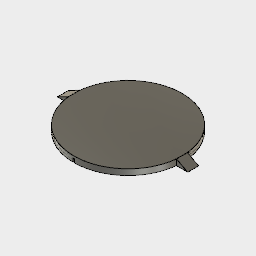
Sand Hopper Lid v1 (Autodesk Fusion 360 design; units mm, degrees)
Autodesk Fusion 360 part; units mm, degrees
sketch "Sketch1" plane through (0, 0, 0) normal (0, 0, 1) x (1, 0, 0)
  circle A0 centre (0, 0) radius 72.5
  dimension "d1" = 145
  constraint coincident A0.centre origin
  measures "d1" diameter of A0
extrude "Extrude1" add sketch "Sketch1" along normal blind 2
sketch "Sketch2" plane through (0, 0, 2) normal (0, 0, 1) x (-1, 0, 0)
  circle A0 centre (0, 0) radius 72.5
  circle A1 centre (0, 0) radius 73.5
  circle A2 centre (0, 0) radius 72.5
  dimension "d4" = 147
  constraint coincident A0.centre A1.centre
  measures "d4" diameter of A1
extrude "Extrude2" add sketch "Sketch2" against normal blind 8
sketch "Sketch3" plane through (0, 0, 0) normal (0, 1, 0) x (1, 0, 0)
  line L0 (73.5, 6) -> (-73.5, 6)
  line L1 (-73.5, -2) -> (73.5, -2)
  line L2 (-72.5, 6) -> (72.5, 6)
  line L3 (-72.5, 0) -> (72.5, 0)
  line L4 (-72.5, 6) -> (-72.5, 3)
  line L5 (-72.5, 3) -> (-69, 3)
  line L6 (-69, 3) -> (-72.5, 6)
  constraint perpendicular L0 L4
  constraint perpendicular L4 L5
revolve "Revolve1" add sketch "Sketch3" angle 360 about axis through (0, 0, 1.75) along (0, 0, 1)
sketch "Sketch4" plane through (0, 0, -6) normal (0, 0, -1) x (1, 0, 0)
  circle A0 centre (0, 0) radius 73.5
  circle A1 centre (0, 0) radius 73.5
  circle A2 centre (0, 0) radius 69
  line L0 (-1, 73.511) -> (-1, 68.9928)
  line L1 (1, 73.4958) -> (1, 68.9928)
  circle A3 centre (0, 0) radius 73.5
  circle A4 centre (0, 0) radius 73.5
  arc A5 (-1, 73.511) -> (1, 73.4958) centre (2.2368, 367.7275) ccw
  line L2 (-1, -68.9928) -> (-1, -73.4932)
  circle A6 centre (0, 0) radius 69
  circle A7 centre (0, 0) radius 69
  line L3 (1, -68.9928) -> (1, -73.4932)
  constraint tangent A4 A5
  constraint coincident A2 A0.centre
  constraint coincident A1
extrude "Extrude3" cut sketch "Sketch4" against normal blind 5 contours A0 A1 A2 A3 A4 L2 A6 A7 L3 | A0 A1 A2 L0 L1 A3 A4 A6 A7
sketch "Sketch5" plane through (0, 0, -6) normal (0, 0, -1) x (1, 0, 0)
  line L0 (1, 73.4932) -> (1, 72.4931)
  arc A0 (1, -72.4931) -> (1, 72.4931) centre (0, 0) ccw
  line L1 (1, -72.4931) -> (1, -73.4932)
  arc A1 (1, -73.4932) -> (1, 73.4932) centre (0, 0) ccw
  arc A2 (1, -73.4932) -> (1, 73.4932) centre (0, 0) ccw
  line L2 (73.1163, -7.5) -> (88.5, -7.5)
  line L3 (73.1163, 7.5) -> (88.5, 7.5)
  line L4 (88.5, -7.5) -> (88.5, 7.5)
  constraint coincident A2 A0.centre
  constraint coincident A2
  constraint perpendicular L3 L4
extrude "Extrude4" add sketch "Sketch5" against normal blind 8 contours A1 A2 L2 L3 L4
sketch "Sketch6" plane through (0, -7.5, 0) normal (0, -1, 0) x (1, 0, 0)
  line L0 (73.1163, -6) -> (88.5, -6)
  line L1 (88.5, -6) -> (88.5, 2)
  line L2 (88.5, 2) -> (73.1163, 2)
  line L3 (73.1163, 2) -> (73.1163, -6)
  line L4 (88.5, -6) -> (73.1163, 2)
  line L5 (73.1163, 2) -> (88.5, 2)
  line L6 (88.5, -6) -> (88.5, 2)
extrude "Extrude5" cut sketch "Sketch6" against normal blind 15 contours L1 L2 L4 L5 L6
sketch "Sketch7" plane through (0, 0, 2) normal (0, 0, 1) x (-1, 0, 0)
  line L0 (-73.1163, 7.5) -> (-73.1163, -7.5)
  arc A0 (-73.1163, -7.5) -> (-73.1163, 7.5) centre (0, 0) ccw
  line L1 (-73.1163, 7.5) -> (-88.5, 7.5)
  line L2 (-88.5, 7.5) -> (-88.5, -7.5)
  line L3 (-88.5, -7.5) -> (-73.1163, -7.5)
  line L4 (-73.1163, -7.5) -> (-73.1163, 7.5)
  line L5 (0, 10) -> (0, -11.5199)
  line L6 (73.1163, 7.5) -> (88.5, 7.5)
  line L7 (88.5, 7.5) -> (88.5, -7.5)
  line L8 (88.5, -7.5) -> (73.1163, -7.5)
  line L9 (73.1163, 7.5) -> (73.1163, -7.5)
  constraint vertical L5
extrude "Extrude6" add sketch "Sketch7" against normal blind 8 contours A0 L6 L7 L8
sketch "Sketch8" plane through (0, -7.5, 0) normal (0, -1, 0) x (1, 0, 0)
  line L0 (-73.1163, 2) -> (-88.5, 2)
  line L1 (-88.5, 2) -> (-88.5, -6)
  line L2 (-88.5, -6) -> (-73.1163, -6)
  line L3 (-73.1163, -6) -> (-73.1163, 2)
  line L4 (-88.5, -6) -> (-73.1163, 2)
  line L5 (-88.5, 2) -> (-88.5, -6)
  line L6 (-88.5, 2) -> (-73.1163, 2)
extrude "Extrude7" cut sketch "Sketch8" against normal blind 15 contours L0 L1 L4 L5 L6
